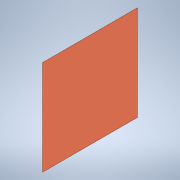
# Autodesk Inventor part: flag
Saved by Autodesk Inventor 2020.2 (Build 242310000, 310)
## iProperties
Created: 2020-03-22
Part Number: flag
Material: PVC, Unplasticized
Document SubType Name: Modeling
Designer: agmle
Density: 1.29 g/cm^3
Appearance: Smooth - Light Orange
Author: agmle
Autodesk Inventor part; units mm, degrees
ref_plane "YZ Plane" through (0, 0, 0) normal (1, 0, 0) x (0, 1, 0)
ref_plane "XZ Plane" through (0, 0, 0) normal (0, 1, 0) x (-1, 0, 0)
ref_plane "XY Plane" through (0, 0, 0) normal (0, 0, 1) x (1, 0, 0)
sketch "Sketch1" plane through (0, 0, 0) normal (1, 0, 0) x (0, 1, 0)
  line L0 (0, 0) -> (596.9, 0)
  line L1 (596.9, 0) -> (596.9, -596.9)
  line L2 (596.9, -596.9) -> (0, -596.9)
  line L3 (0, -596.9) -> (0, 0)
  dimension "d0" = 596.9
  constraints: 8 end point, 2 parallel, 2 perpendicular, 1 horizontal
  measures "d0" distance of L0.start L0.end
extrude "Extrusion1" add sketch "Sketch1" along normal blind 0.3175
body "Solid1"
